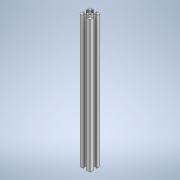
# Autodesk Inventor part: Profilé
Saved by Autodesk Inventor 2020 (Build 240168000, 168)
## iProperties
Created: 2019-11-28
Part Number: Profilé
Material: Générique
Document SubType Name: Modeling
Designer: erwan
Density: 1 g/cm^3
Appearance: Par défaut
Author: erwan
Autodesk Inventor part; units mm, degrees
ref_plane "YZ Plane" through (0, 0, 0) normal (1, 0, 0) x (0, 1, 0)
ref_plane "XZ Plane" through (0, 0, 0) normal (0, 1, 0) x (-1, 0, 0)
ref_plane "XY Plane" through (0, 0, 0) normal (0, 0, 1) x (1, 0, 0)
sketch "Esquisse1" plane through (0, 0, 0) normal (0, 1, 0) x (-1, 0, 0)
  circle A0 centre (0, 0) radius 2.5
  line L0 (0, -4) -> (3, -4)
  line L1 (4, 0) -> (4, -3)
  line L2 (4, 0) -> (4, 3)
  line L3 (0, 4) -> (3, 4)
  line L4 (0, 4) -> (-3, 4)
  line L5 (-4, 0) -> (-4, -3)
  line L6 (-4, 0) -> (-4, 3)
  line L7 (0, -4) -> (-3, -4)
  line L8 (5.5, -6.5) -> (3, -4)
  line L9 (6.5, -5.5) -> (4, -3)
  line L10 (5.5, 6.5) -> (3, 4)
  line L11 (6.5, 5.5) -> (4, 3)
  line L12 (-5.5, 6.5) -> (-3, 4)
  line L13 (-6.5, 5.5) -> (-4, 3)
  line L14 (-6.5, -5.5) -> (-4, -3)
  line L15 (-3, -4) -> (-5.5, -6.5)
  line L16 (5.5, -6.5) -> (5.5, -8.25)
  line L17 (5.5, -8.25) -> (3, -8.25)
  line L18 (-5.5, -6.5) -> (-5.5, -8.25)
  line L19 (-5.5, -8.25) -> (-3, -8.25)
  line L20 (-6.5, -5.5) -> (-8.25, -5.5)
  line L21 (-8.25, -5.5) -> (-8.25, -3)
  line L22 (-6.5, 5.5) -> (-8.25, 5.5)
  line L23 (-8.25, 5.5) -> (-8.25, 3)
  line L24 (-5.5, 6.5) -> (-5.5, 8.25)
  line L25 (-5.5, 8.25) -> (-3, 8.25)
  line L26 (5.5, 6.5) -> (5.5, 8.25)
  line L27 (5.5, 8.25) -> (3, 8.25)
  line L28 (6.5, 5.5) -> (8.25, 5.5)
  line L29 (8.25, 5.5) -> (8.25, 3)
  line L30 (6.5, -5.5) -> (8.25, -5.5)
  line L31 (8.25, -5.5) -> (8.25, -3)
  line L32 (3, -8.25) -> (3, -10)
  line L33 (-3, -8.25) -> (-3, -10)
  line L34 (-8.25, -3) -> (-10, -3)
  line L35 (-8.25, 3) -> (-10, 3)
  line L36 (-3, 8.25) -> (-3, 10)
  line L37 (3, 8.25) -> (3, 10)
  line L38 (8.25, 3) -> (10, 3)
  line L39 (8.25, -3) -> (10, -3)
  line L40 (3, 10) -> (10, 10)
  line L41 (10, 10) -> (10, 3)
  line L42 (10, -3) -> (10, -10)
  line L43 (10, -10) -> (3, -10)
  line L44 (-3, -10) -> (-10, -10)
  line L45 (-10, -10) -> (-10, -3)
  line L46 (-10, 3) -> (-10, 10)
  line L47 (-3, 10) -> (-10, 10)
  dimension "d4" = 5
  dimension "d5" = 3
  dimension "d6" = 3
  dimension "d7" = 3
  dimension "d8" = 3
  dimension "d9" = 3
  dimension "d10" = 3
  dimension "d11" = 3
  dimension "d12" = 3
  dimension "d17" = 1.75
  dimension "d18" = 2.5
  dimension "d19" = 1.75
  dimension "d20" = 1.75
  dimension "d21" = 1.75
  dimension "d22" = 1.75
  constraints: 96 end point, 13 perpendicular, 8 point on line, 5 horizontal, 4 vertical, 3 parallel, 1 centre point, 1 coincident
  measures "d4" diameter of A0
  measures "d5" distance of L0.start L0.end
  measures "d6" distance of L1.start L1.end
  measures "d7" distance of L1.start L2.end
  measures "d8" distance of L3.start L3.end
  measures "d9" distance of L3.start L4.end
  measures "d10" distance of L5.start L5.end
  measures "d11" distance of L5.start L6.end
  measures "d12" distance of L0.start L7.end
  measures "d17" distance of L8.start L16.end
  measures "d18" distance of L16.end L17.end
  measures "d19" distance of L14.start L20.end
  measures "d20" distance of L13.start L22.end
  measures "d21" distance of L12.start L24.end
  measures "d22" distance of L11.start L28.end
extrude "Extrusion1" add sketch "Esquisse1" along normal blind 250
fillet "Congé1" radius 1.5 4 edges at (-10, 125, 10) (10, 125, 10) (-10, 125, -10) (10, 125, -10)
